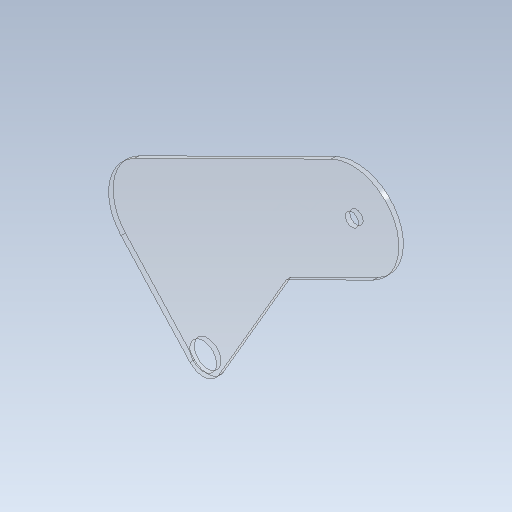
# Autodesk Inventor part: ダンパーガード
Saved by Autodesk Inventor 2020.2 (Build 242310000, 310)
## iProperties
Created: 2020-03-26
Part Number: ダンパーガード
Material: ポリカーボネート、クリア
Document SubType Name: Modeling
Designer: aoyam
Density: 1.2 g/cm^3
Appearance: ポリカーボネート - クリア
Mass: 1.92229 g
Surface Area: 34.1248 cm^2
Volume: 1.6019 cm^3
Author: aoyam
Autodesk Inventor part; units mm, degrees
ref_plane "YZ Plane" through (0, 0, 0) normal (1, 0, 0) x (0, 1, 0)
ref_plane "XZ Plane" through (0, 0, 0) normal (0, 1, 0) x (-1, 0, 0)
ref_plane "XY Plane" through (0, 0, 0) normal (0, 0, 1) x (1, 0, 0)
sketch "スケッチ1" plane through (0, 0, 0) normal (0, 0, 1) x (1, 0, 0)
  circle A0 centre (23.2, 20.8573) radius 3
  circle A1 centre (56.5578, 64) radius 1.5
  line L0 (23.2, 20.8573) -> (56.5578, 64)
  line L1 (23.2, 20.8573) -> (56.5578, 64) construction
  circle A2 centre (56.5578, 64) radius 1.5
  line L2 (23.2, 20.8573) -> (12.5297, 42.1181)
  line L3 (12.5297, 42.1181) -> (56.5578, 64) construction
  line L4 (17.2029, 32.7153) -> (61.231, 54.5973)
  line L5 (51.8846, 73.4027) -> (7.8565, 51.5208)
  arc A3 (7.8565, 51.5208) -> (17.2029, 32.7153) centre (12.5297, 42.1181) ccw
  arc A4 (61.231, 54.5973) -> (51.8846, 73.4027) centre (56.5578, 64) ccw
  circle A5 centre (23.2, 20.8573) radius 4
  line L6 (4.7893, 35.0232) -> (20.2513, 18.1545)
  line L7 (41.8337, 44.9568) -> (26.6583, 18.8472)
  point P0 (0, 0)
  point P1 (0, 0)
  point P2 (39.8789, 42.4286)
  point P3 (34.5437, 53.059)
  point P4 (26.2844, 23.4042)
  point P5 (20.1698, 18.2461)
  point P6 (25.5392, 22.7356)
  point P7 (21.8543, 23.5385)
  point P8 (21.4058, 24.4323)
  point P9 (25.6467, 24.0217)
  point P10 (25.035, 23.2306)
  dimension "d6" = 3
  dimension "d7" = 21
  dimension "d8" = 8
  constraints: 20 end point, 7 point on circle, 7 tangent, 6 centre point, 3 point on line, 2 equal length, 2 midpoint, 3 other
  measures "d6" diameter of A2
  measures "d7" diameter of A4
  measures "d8" diameter of A5
extrude "押し出し1" add sketch "スケッチ1" along normal blind 1 contours A0 L0 A5 L2 | A0 L2 A5 L0 | A5 L2 L4 L0 | L0 L7 A5 | A5 L6 A3 L4 L2 | L4 A3 L5 A4
